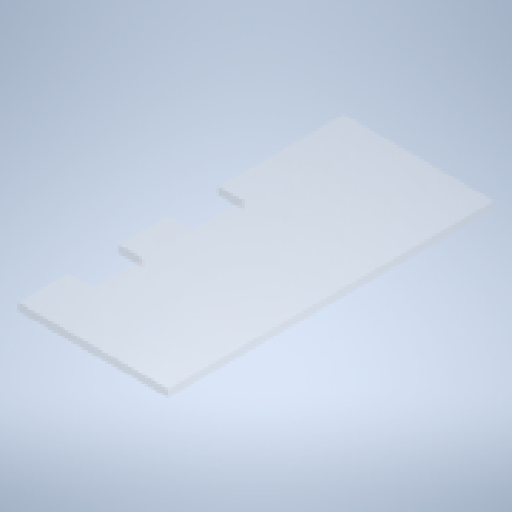
# Autodesk Inventor part: 발받침대받침옆판2
Saved by Autodesk Inventor 2024 (Build 280153000, 153)
## iProperties
Created: 2024-04-10
Part Number: 발받침대받침옆판2
Material: PMMA 플라스틱
Document SubType Name: Modeling
Designer: kkamin5
Mass: 39.204 g
Surface Area: 149 cm^2
Volume: 33 cm^3
Density: 1.188 g/cm^3
Appearance: 폴리카보네이트 - 선명
Author: kkamin5
Autodesk Inventor part; units mm, degrees
ref_plane "YZ Plane" through (0, 0, 0) normal (1, 0, 0) x (0, 1, 0)
ref_plane "XZ Plane" through (0, 0, 0) normal (0, 1, 0) x (-1, 0, 0)
ref_plane "XY Plane" through (0, 0, 0) normal (0, 0, 1) x (1, 0, 0)
sketch "스케치1" plane through (0, 0, 0) normal (0, 1, 0) x (-1, 0, 0)
  line L0 (30, 65) -> (-30, 65)
  line L1 (-30, 65) -> (-30, -65)
  line L2 (-30, -65) -> (30, -65)
  line L3 (30, -65) -> (30, 65)
  point P0 (0, 0)
  dimension "d0" = 130
  dimension "d1" = 60
  dimension "d2" = 30
  dimension "d3" = 65
  constraints: 8 end point, 2 parallel, 1 horizontal, 1 perpendicular
  measures "d0" distance of L0.end L1.end
  measures "d1" distance of L1.end L2.end
  measures "d2" distance from line of point (0, 0) L3
  measures "d3" distance from line of point (0, 0) L0
extrude "돌출1" add sketch "스케치1" along normal blind 3
sketch "스케치2" plane through (0, 3, 0) normal (0, 1, 0) x (1, 0, 0)
  line L0 (-30, 65) -> (-30, -65) projected
  line L1 (-10, 39) -> (-30, 39)
  line L2 (-30, 39) -> (-30, 13)
  line L3 (-30, 13) -> (-10, 13)
  line L4 (-10, 13) -> (-10, 39)
  line L5 (-10, -13) -> (-30, -13)
  line L6 (-30, -13) -> (-30, -39)
  line L7 (-30, -39) -> (-10, -39)
  line L8 (-10, -39) -> (-10, -13)
  line L9 (-30, -65) -> (30, -65) projected
  point P0 (0, 0)
  point P1 (-30, -13)
  dimension "d6" = 26
  dimension "d7" = 26
  dimension "d8" = 26
  dimension "d9" = 26
  dimension "d10" = 20
  constraints: 16 end point, 4 parallel, 3 point on line, 2 horizontal, 2 perpendicular
  measures "d6" distance between parallel lines of L7 L9
  measures "d7" distance between parallel lines of L7 L5
  measures "d8" distance between parallel lines of L5 L3
  measures "d9" distance between parallel lines of L3 L1
  measures "d10" distance between parallel lines of L0 L8
extrude "돌출2" cut sketch "스케치2" against normal blind 10
equation "\"d3\" = 0.5 * d0"
equation "\"d7\" = d6"
equation "\"d8\" = d7"
equation "\"d9\" = d8"
